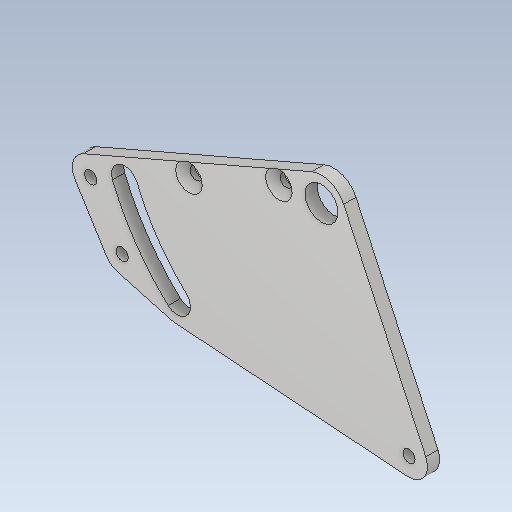
# Autodesk Inventor part: 中間外フレーム2
Saved by Autodesk Inventor 2020 (Build 240168000, 168)
## iProperties
Created: 2019-11-12
Part Number: 中間外フレーム2
Material: アルミニウム 2014-T4
Document SubType Name: Modeling
Designer: tanjihayato
Density: 2.8 g/cm^3
Appearance: サテン
Mass: 10.3329 g
Surface Area: 69.2935 cm^2
Volume: 3.69031 cm^3
Author: tanjihayato
Autodesk Inventor part; units mm, degrees
ref_plane "YZ Plane" through (0, 0, 0) normal (1, 0, 0) x (0, 1, 0)
ref_plane "XZ Plane" through (0, 0, 0) normal (0, 1, 0) x (-1, 0, 0)
ref_plane "XY Plane" through (0, 0, 0) normal (0, 0, 1) x (1, 0, 0)
sketch "スケッチ1" plane through (0, 0, 0) normal (0, 0, 1) x (1, 0, 0)
  circle A0 centre (0, 0) radius 20.55 construction
  circle A1 centre (-21.6908, -16.4118) radius 19.1 construction
  circle A2 centre (25.3202, -9.9362) radius 19.1 construction
  circle A3 centre (-50.601, 30.8143) radius 1.5
  circle A4 centre (5.9362, 53.5882) radius 1.5
  circle A5 centre (27.3908, 10.6821) radius 1.5
  circle A6 centre (-42.8914, 18.3887) radius 1.5
  circle A7 centre (-21.6908, -16.4118) radius 4.025
  circle A8 centre (25.3202, -9.9362) radius 4.025
  circle A9 centre (0, 0) radius 4
  line L0 (-17.8785, -18.8026) -> (-30.4168, -38.7963) construction
  arc A10 (-17.8785, -18.8026) -> (-19.2493, -12.6317) centre (-21.6908, -16.4118) ccw construction
  line L1 (-19.2493, -12.6317) -> (-39.0737, 0.1727) construction
  line L2 (37.1409, -30.8522) -> (21.8866, -12.8448) construction
  arc A11 (22.3659, -6.5417) -> (21.8866, -12.8448) centre (25.3202, -9.9362) ccw construction
  line L3 (22.3659, -6.5417) -> (40.1678, 8.9519) construction
  line L4 (-21.6908, -16.4118) -> (-99.9742, 13.5882) construction
  line L5 (-105.5257, -16.4118) -> (-21.6908, -16.4118) construction
  line L6 (-21.6908, -16.4118) -> (-101.7113, -41.4118) construction
  line L7 (25.3202, -9.9362) -> (102.5386, -46.4118) construction
  line L8 (110.4743, -16.4118) -> (25.3202, -9.9362) construction
  line L9 (25.3202, -9.9362) -> (108.6869, 8.5882) construction
  line L10 (-18.0583, -13.7557) -> (-31.9879, 5.2949) construction
  line L11 (-17.339, -17.5569) -> (-24.5367, -44.9106) construction
  line L12 (21.5077, -7.5456) -> (34.045, 12.4488) construction
  line L13 (21.0739, -11.4259) -> (31.6059, -41.446) construction
  arc A12 (-24.6176, -40.3201) -> (-19.5065, -44.4166) centre (-20.132, -39.9603) ccw
  circle A13 centre (-20.132, -39.9603) radius 3 construction
  arc A14 (-38.9879, 7.9907) -> (-39.3359, 8.5262) centre (-35.3982, 10.7044) ccw construction
  circle A15 centre (-35.3982, 10.7044) radius 3 construction
  arc A16 (-31.9879, 5.2949) -> (-33.8465, 6.7744) centre (-35.6204, 2.6388) ccw construction
  circle A17 centre (-41.5152, -3.6073) radius 1.5
  line L14 (-33.8465, 6.7744) -> (-56.066, 16.3055) construction
  line L15 (-41.3386, 0.8892) -> (-72.6317, 2.1181) construction
  circle A18 centre (-42.8914, 18.3887) radius 3 construction
  circle A19 centre (-35.3982, 10.7044) radius 1.5
  circle A20 centre (36.7736, 17.5344) radius 1.5
  arc A21 (40.7942, 15.5132) -> (40.1934, 20.4593) centre (36.7736, 17.5344) ccw
  circle A22 centre (25.6508, -33.5339) radius 1.5
  arc A23 (26.2763, -37.9902) -> (30.1508, -33.5178) centre (25.6508, -33.5339) ccw
  circle A24 centre (36.7736, 17.5344) radius 3 construction
  circle A25 centre (25.6508, -33.5339) radius 3 construction
  arc A26 (36.6836, 14.4025) -> (34.045, 12.4488) centre (37.8575, 10.0583) ccw construction
  line L16 (36.6836, 14.4025) -> (64.1968, 21.8369) construction
  line L17 (43.2599, 10.0553) -> (82.9273, 8.8396) construction
  circle A27 centre (27.3908, 10.6821) radius 3 construction
  circle A28 centre (-21.6908, -16.4118) radius 7.025 construction
  circle A29 centre (25.3202, -9.9362) radius 7.025 construction
  arc A30 (40.8593, 15.6483) -> (30.1508, -33.5178) centre (146.4685, -33.1029) ccw
  arc A31 (-24.6176, -40.3201) -> (-39.1827, 8.2484) centre (-145.1158, -49.988) ccw
  arc A32 (-52.2824, 34.9884) -> (-54.1907, 28.1005) centre (-50.601, 30.8143) ccw
  arc A33 (9.356, 56.5132) -> (4.2549, 57.7623) centre (5.9362, 53.5882) ccw
  line L18 (-39.1827, 8.2484) -> (-54.1907, 28.1005)
  line L19 (-52.2824, 34.9884) -> (4.2549, 57.7623)
  line L20 (9.356, 56.5132) -> (40.1934, 20.4593)
  line L21 (-19.5065, -44.4166) -> (26.2763, -37.9902)
  circle A34 centre (-20.132, -39.9603) radius 1.5
  line L22 (-23.8868, -42.4405) -> (-17.339, -17.5569)
  arc A35 (-17.339, -17.5569) -> (-18.0583, -13.7557) centre (-21.6908, -16.4118) ccw
  line L23 (-18.0583, -13.7557) -> (-31.9879, 5.2949)
  arc A36 (-31.9879, 5.2949) -> (-33.8465, 6.7744) centre (-35.6204, 2.6388) ccw
  line L24 (-33.8465, 6.7744) -> (-40.0946, 9.4545)
  line L25 (40.7974, 15.5141) -> (36.6836, 14.4025)
  arc A37 (36.6836, 14.4025) -> (34.045, 12.4488) centre (37.8575, 10.0583) ccw
  line L26 (34.045, 12.4488) -> (21.5077, -7.5456)
  arc A38 (21.5077, -7.5456) -> (21.0739, -11.4259) centre (25.3202, -9.9362) ccw
  line L27 (21.0739, -11.4259) -> (29.592, -35.7057)
  dimension "d0" = 8.05
  dimension "d1" = 8.05
  dimension "d2" = 8
  dimension "d3" = 20.968
  dimension "d4" = 20.968
  dimension "d5" = 17.35
  dimension "d6" = 17.35
  dimension "d7" = 16.877
  dimension "d8" = 16.877
  dimension "d9" = 20.936
  dimension "d10" = 20.936
  dimension "d11" = 9
  dimension "d12" = 6
  dimension "d13" = 9
  dimension "d14" = 6
  dimension "d15" = 9
  dimension "d16" = 20.968
  dimension "d17" = 20.968
  dimension "d18" = 6
  dimension "d19" = 3
  dimension "d20" = 3
  dimension "d21" = 9
  dimension "d22" = 3
  dimension "d23" = 9
  dimension "d24" = 6
  dimension "d25" = 6
  dimension "d26" = 9
  dimension "d27" = 16.877
  dimension "d28" = 3
  dimension "d29" = 3
  dimension "d30" = 9
  dimension "d31" = 9
  dimension "d32" = 3
  constraints: 56 end point, 40 point on circle, 39 centre point, 31 tangent, 14 coincident, 6 point on line, 2 equal length, 1 collinear, 1 concentric
  measures "d0" diameter of A7
  measures "d1" diameter of A8
  measures "d2" diameter of A9
  measures "d3" angle of L5 L4
  measures "d4" angle of L1 L10
  measures "d5" angle of L5 L6
  measures "d6" angle of L0 L11
  measures "d7" angle of L8 L9
  measures "d8" angle of L12 L3
  measures "d9" angle of L8 L7
  measures "d10" angle of L13 L2
  measures "d11" diameter of A12
  measures "d12" diameter of A13
  measures "d13" diameter of A14
  measures "d14" diameter of A15
  measures "d15" diameter of A16
  measures "d17" angle of L15 L14
  measures "d18" diameter of A18
  measures "d19" diameter of A19
  measures "d20" diameter of A20
  measures "d21" diameter of A21
  measures "d22" diameter of A22
  measures "d23" diameter of A23
  measures "d24" diameter of A24
  measures "d25" diameter of A25
  measures "d26" diameter of A26
  measures "d27" angle of L16 L17
  measures "d28" radial gap between concentric circles of A7 A28
  measures "d29" radial gap between concentric circles of A8 A29
  measures "d30" diameter of A32
  measures "d31" diameter of A33
  measures "d32" diameter of A34
sketch "スケッチ2" plane through (0, 0, 0) normal (0, 0, 1) x (1, 0, 0)
  circle A0 centre (-50.601, 30.8143) radius 1.5 projected
  circle A1 centre (-42.8914, 18.3887) radius 1.5 projected
  circle A2 centre (5.9362, 53.5882) radius 1.5 projected
  circle A3 centre (27.3908, 10.6821) radius 1.5 projected
  arc A4 (-52.3846, 34.9457) -> (-54.4248, 28.4418) centre (-50.601, 30.8143) ccw
  arc A5 (-46.7151, 16.0162) -> (-43.3819, 13.9155) centre (-42.8914, 18.3887) ccw
  arc A6 (11.384, 56.1025) -> (3.5581, 59.0968) centre (5.9362, 53.5882) ccw
  arc A7 (26.9003, 6.2089) -> (31.4766, 12.5678) centre (27.3908, 10.6821) ccw
  line L0 (-46.7151, 16.0162) -> (-54.4248, 28.4418)
  line L1 (-52.3846, 34.9457) -> (3.5581, 59.0968)
  line L2 (11.384, 56.1025) -> (31.4766, 12.5678)
  line L3 (26.9003, 6.2089) -> (-43.3819, 13.9155)
  circle A8 centre (5.9362, 53.5882) radius 4.025
  point P0 (0, 0)
  dimension "d33" = 3
  dimension "d34" = 3
  dimension "d35" = 4.5
  dimension "d36" = 3
  dimension "d39" = 8.05
  constraints: 8 end point, 8 point on circle, 8 tangent, 5 centre point, 1 coincident
  measures "d33" radial gap between concentric circles of A0 A4
  measures "d34" radial gap between concentric circles of A1 A5
  measures "d35" radial gap between concentric circles of A2 A6
  measures "d36" radial gap between concentric circles of A3 A7
  measures "d39" diameter of A8
extrude "押し出し1" add sketch "スケッチ2" along normal blind 3 contours L1 A6 L2 A7 L3 A5 L0 A4
sketch "スケッチ3" plane through (0, 0, 3) normal (0, 0, 1) x (1, 0, 0)
  circle A0 centre (5.9362, 53.5882) radius 4.025 projected
  circle A1 centre (27.3908, 10.6821) radius 1.5 projected
  circle A2 centre (-42.8914, 18.3887) radius 1.5 projected
  circle A3 centre (-50.601, 30.8143) radius 1.5 projected
  line L0 (-54.4248, 28.4418) -> (-46.7151, 16.0162) projected
  arc A4 (-46.7151, 16.0162) -> (-43.3819, 13.9155) centre (-42.8914, 18.3887) ccw projected
  line L1 (-43.3819, 13.9155) -> (26.9003, 6.2089) projected
  arc A5 (26.9003, 6.2089) -> (31.4766, 12.5678) centre (27.3908, 10.6821) ccw projected
  line L2 (31.4766, 12.5678) -> (11.384, 56.1025) projected
  arc A6 (11.384, 56.1025) -> (3.5581, 59.0968) centre (5.9362, 53.5882) ccw projected
  line L3 (3.5581, 59.0968) -> (-52.3846, 34.9457) projected
  arc A7 (-52.3846, 34.9457) -> (-54.4248, 28.4418) centre (-50.601, 30.8143) ccw projected
  circle A8 centre (5.9362, 53.5882) radius 6
  circle A9 centre (-26.5254, 42.8418) radius 1.5
  circle A10 centre (-4.491, 52.3543) radius 1.5
  circle A11 centre (-4.491, 52.3543) radius 4.5 construction
  point P0 (0, 0)
  dimension "d40" = 12
  dimension "d41" = 3
  dimension "d42" = 3
  dimension "d43" = 3
  dimension "d44" = 3
  dimension "d45" = 24
  dimension "d46" = 9
  constraints: 4 centre point, 2 coincident, 1 tangent
  measures "d40" diameter of A8
  measures "d41" diameter of A9
  measures "d42" diameter of A10
  measures "d43" distance from line of L3 A10.centre
  measures "d44" distance from line of L3 A9.centre
  measures "d45" distance of A9.centre A10.centre
  measures "d46" diameter of A11
extrude "押し出し2" cut sketch "スケッチ3" against normal blind 10 contours A9 | A10
chamfer "面取り1" distance 1.75 angle 45 2 edges at (-5.991, 52.3543, 3) (-28.0254, 42.8418, 3)
sketch "スケッチ4" plane through (0, 0, 3) normal (0, 0, 1) x (1, 0, 0)
  circle A0 centre (127.6431, 30.2622) radius 1.5
  circle A1 centre (5.9362, 53.5882) radius 1.5
  line L0 (5.9362, 53.5882) -> (127.6431, 30.2622) construction
  circle A2 centre (5.9362, 53.5882) radius 4.025
  circle A3 centre (127.6431, 30.2622) radius 4.025
  arc A4 (127.2517, 23.2481) -> (128.9655, 37.1616) centre (127.6431, 30.2622) ccw
  line L1 (12.8357, 52.2659) -> (13.4004, 55.2122)
  line L2 (15.4628, 54.817) -> (26.0698, 52.7841)
  line L3 (28.1322, 52.3888) -> (27.5675, 49.4424)
  line L4 (14.8981, 51.8706) -> (25.5051, 49.8377)
  line L5 (120.7437, 31.5845) -> (121.3084, 34.5309)
  line L6 (119.246, 34.9262) -> (108.639, 36.9591)
  line L7 (106.5765, 37.3543) -> (106.0119, 34.408)
  line L8 (108.0743, 34.0127) -> (118.6813, 31.9798)
  circle A5 centre (19.3546, 46.4346) radius 3
  circle A6 centre (112.5307, 28.5767) radius 3
  line L9 (7.2586, 60.4876) -> (128.9655, 37.1616)
  arc A7 (17.9263, 42.1672) -> (21.5465, 42.5045) centre (19.3546, 46.4346) ccw
  arc A8 (109.041, 25.7356) -> (112.28, 24.0837) centre (112.5307, 28.5767) ccw
  line L10 (3.7066, 46.9264) -> (17.9263, 42.1672)
  line L11 (112.28, 24.0837) -> (127.2517, 23.2481)
  circle A9 centre (19.3546, 46.4346) radius 1.5
  circle A10 centre (112.5307, 28.5767) radius 1.5
  line L12 (32.3442, 48.5269) -> (21.5465, 42.5045)
  line L13 (109.041, 25.7356) -> (101.2351, 35.3235)
  line L14 (32.3442, 48.5269) -> (101.2351, 35.3235)
  arc A11 (108.639, 36.9591) -> (106.5765, 37.3543) centre (107.6078, 37.1567) ccw
  arc A12 (106.0119, 34.408) -> (108.0743, 34.0127) centre (107.0431, 34.2103) ccw
  arc A13 (121.3084, 34.5309) -> (119.246, 34.9262) centre (120.2772, 34.7285) ccw
  arc A14 (118.6813, 31.9798) -> (120.7437, 31.5845) centre (119.7125, 31.7821) ccw
  arc A15 (28.1322, 52.3888) -> (26.0698, 52.7841) centre (27.101, 52.5864) ccw
  arc A16 (25.5051, 49.8377) -> (27.5675, 49.4424) centre (26.5363, 49.64) ccw
  arc A17 (15.4628, 54.817) -> (13.4004, 55.2122) centre (14.4316, 55.0146) ccw
  arc A18 (12.8357, 52.2659) -> (14.8981, 51.8706) centre (13.8669, 52.0682) ccw
  line L15 (5.9362, 53.5882) -> (-35.9404, 22.842) construction
  circle A19 centre (-35.9404, 22.842) radius 1.5
  arc A20 (-37.7159, 25.2602) -> (-34.165, 20.4238) centre (-35.9404, 22.842) ccw
  line L16 (-37.7159, 25.2602) -> (-0.9595, 52.247)
  line L17 (-34.165, 20.4238) -> (2.5914, 47.4106)
  arc A21 (7.2586, 60.4876) -> (-0.9595, 52.247) centre (5.9362, 53.5882) ccw
  arc A22 (2.5914, 47.4106) -> (3.7066, 46.9264) centre (5.9362, 53.5882) ccw
  circle A23 centre (0, 0) radius 10.1 construction
  circle A24 centre (25.3202, -9.9362) radius 17.1 construction
  circle A25 centre (110.4743, -16.4118) radius 28.1 construction
  circle A26 centre (62.4131, -12.7569) radius 20.1 construction
  circle A27 centre (-21.6908, -16.4118) radius 17.1 construction
  circle A28 centre (-105.5257, -16.4118) radius 28.1 construction
  line L18 (-170.915, -81.4118) -> (490.0044, -81.4118)
  line L19 (-105.5257, -16.4118) -> (-21.6908, -16.4118) construction
  line L20 (110.4743, -16.4118) -> (25.3202, -9.9362) construction
  line L21 (110.4743, -16.4118) -> (104.1501, -0.632)
  line L22 (104.1501, -0.632) -> (95.5937, 20.7173) construction
  line L23 (95.5937, 20.7173) -> (70.4743, -10.4118) construction
  line L24 (70.4743, -10.4118) -> (110.4743, -16.4118) construction
  line L25 (-137.6819, 53.5882) -> (165.8186, 53.5882)
  line L26 (25.3202, -9.9362) -> (108.6869, 8.5882) construction
  line L27 (25.3202, -9.9362) -> (102.5386, -46.4118) construction
  line L28 (25.3202, -9.9362) -> (5.9362, 53.5882) construction
  line L29 (5.9362, 53.5882) -> (127.6431, 30.2622)
  line L30 (127.6431, 30.2622) -> (110.4743, -16.4118) construction
  line L31 (102.5386, -46.4118) -> (118.0681, 0.8329) construction
  line L32 (118.0681, 0.8329) -> (5.9362, 53.5882) construction
  line L33 (108.6869, 8.5882) -> (129.8583, 53.5882) construction
  line L34 (129.8583, 53.5882) -> (5.9362, 53.5882) construction
  line L35 (119.2726, 31.0882) -> (366.4441, 68.5882) construction
  line L36 (119.0587, 6.9252) -> (362.0213, 65.8249) construction
  line L37 (110.3034, -22.7894) -> (351.0624, 44.5537) construction
  line L38 (127.6431, 30.2622) -> (4.1927, 19.4617) construction
  circle A29 centre (80.4743, 23.124) radius 3 construction
  circle A30 centre (80.4743, 23.124) radius 1.5
  arc A31 (79.801, 27.5733) -> (76.162, 24.4099) centre (80.4743, 23.124) ccw
  circle A32 centre (70.4743, -10.4118) radius 1.5
  arc A33 (66.162, -9.1259) -> (69.4242, -14.7876) centre (70.4743, -10.4118) ccw
  circle A34 centre (150.4743, 0.5882) radius 1.5
  arc A35 (152.5623, -3.3981) -> (154.0408, 3.3323) centre (150.4743, 0.5882) ccw
  circle A36 centre (127.6431, 30.2622) radius 1.5
  arc A37 (131.2816, 32.9102) -> (126.9698, 34.7115) centre (127.6431, 30.2622) ccw
  circle A38 centre (110.4743, -16.4118) radius 5
  arc A39 (108.6075, -24.1909) -> (114.1862, -23.4986) centre (110.4743, -16.4118) ccw
  line L39 (76.162, 24.4099) -> (66.162, -9.1259)
  line L40 (69.4242, -14.7876) -> (108.6075, -24.1909)
  line L41 (114.1862, -23.4986) -> (152.5623, -3.3981)
  line L42 (154.0408, 3.3323) -> (131.2097, 33.0062)
  line L43 (126.9698, 34.7115) -> (79.801, 27.5733)
  circle A40 centre (-145.5257, 0.5882) radius 1.5
  arc A41 (-149.0922, 3.3323) -> (-147.6136, -3.3981) centre (-145.5257, 0.5882) ccw
  circle A42 centre (-105.5257, -16.4118) radius 5
  arc A43 (-109.2375, -23.4986) -> (-103.6588, -24.1909) centre (-105.5257, -16.4118) ccw
  circle A44 centre (-65.5257, -10.4118) radius 1.5
  arc A45 (-64.4756, -14.7876) -> (-61.2133, -9.1259) centre (-65.5257, -10.4118) ccw
  circle A46 centre (0, 0) radius 20.05 construction
  circle A47 centre (110.4743, -16.4118) radius 30.1 construction
  circle A48 centre (62.4131, -12.7569) radius 22.1 construction
  circle A49 centre (25.3202, -9.9362) radius 19.1 construction
  circle A50 centre (0, 0) radius 12.1 construction
  circle A51 centre (-21.6908, -16.4118) radius 19.1 construction
  circle A52 centre (-105.5257, -16.4118) radius 30.1 construction
  circle A53 centre (0, 0) radius 20.55 construction
  circle A54 centre (95.5937, 20.7173) radius 4.025 construction
  circle A55 centre (95.5937, 20.7173) radius 6.025 construction
  circle A56 centre (-75.5257, 23.124) radius 1.5
  arc A57 (-71.2133, 24.4099) -> (-74.8523, 27.5733) centre (-75.5257, 23.124) ccw
  circle A58 centre (-122.6945, 30.2622) radius 1.5
  arc A59 (-122.0212, 34.7115) -> (-126.261, 33.0062) centre (-122.6945, 30.2622) ccw
  line L44 (-126.261, 33.0062) -> (-149.0922, 3.3323)
  line L45 (-147.6136, -3.3981) -> (-109.2375, -23.4986)
  line L46 (-103.6588, -24.1909) -> (-64.4756, -14.7876)
  line L47 (-61.2133, -9.1259) -> (-71.2133, 24.4099)
  line L48 (-74.8523, 27.5733) -> (-122.0212, 34.7115)
  circle A60 centre (14, -17.4118) radius 2.2921 construction
  circle A61 centre (-14, -17.4118) radius 2.2921 construction
  circle A62 centre (-14, -17.4118) radius 14 construction
  circle A63 centre (14, -17.4118) radius 14 construction
  line L49 (-170.6512, -31.4118) -> (202.8656, -31.4118)
  line L50 (5.9362, 53.5882) -> (-42.2529, 34.177) construction
  line L51 (5.9362, 53.5882) -> (-29.4045, 15.5091) construction
  circle A64 centre (5.9362, 53.5882) radius 1.5
  arc A65 (9.9611, 55.6008) -> (4.2549, 57.7623) centre (5.9362, 53.5882) ccw
  line L52 (-21.6908, -16.4118) -> (-99.9742, 13.5882) construction
  line L53 (-21.6908, -16.4118) -> (-101.7113, -41.4118) construction
  line L54 (9.9611, 55.6008) -> (31.4156, 12.6947)
  circle A66 centre (-50.601, 30.8143) radius 1.5
  arc A67 (-52.2824, 34.9884) -> (-54.4248, 28.4418) centre (-50.601, 30.8143) ccw
  line L55 (4.2549, 57.7623) -> (-52.2824, 34.9884)
  line L56 (-54.4248, 28.4418) -> (-46.7151, 16.0162)
  circle A68 centre (27.3908, 10.6821) radius 3 construction
  circle A69 centre (-84.8661, 5.2713) radius 4.5 construction
  circle A70 centre (-132.0174, -1.9813) radius 4.5 construction
  line L57 (-132.7015, 2.4664) -> (-85.5502, 9.719) construction
  arc A71 (26.9003, 6.2089) -> (31.4156, 12.6947) centre (27.3908, 10.6821) ccw
  arc A72 (-46.7151, 16.0162) -> (-43.3819, 13.9155) centre (-42.8914, 18.3887) ccw
  line L58 (-43.3819, 13.9155) -> (26.9003, 6.2089)
  circle A73 centre (-42.2529, 34.177) radius 3 construction
  circle A74 centre (25.3202, -9.9362) radius 4.025 construction
  circle A75 centre (-21.6908, -16.4118) radius 4.025 construction
  circle A76 centre (-42.8914, 18.3887) radius 1.5
  circle A77 centre (27.3908, 10.6821) radius 1.5
  circle A78 centre (-57.813, 39.7705) radius 4.5 construction
  circle A79 centre (-99.304, 63.3152) radius 4.5 construction
  line L59 (5.9362, 53.5882) -> (-35.9404, 22.842) construction
  circle A80 centre (-58.0056, -24.4791) radius 20.1 construction
  circle A81 centre (-58.0056, -24.4791) radius 22.1 construction
  line L60 (-53.3261, 39.4281) -> (-56.2797, 0.7243) construction
  circle A82 centre (-42.2529, 34.177) radius 4.5
  dimension "d169" = 9
  dimension "d170" = 9
  dimension "d185" = 9
  dimension "d52" = 8.05
  dimension "d53" = 8.05
  dimension "d54" = 3
  dimension "d55" = 3
  dimension "d56" = 15
  dimension "d57" = 3
  dimension "d58" = 15
  dimension "d59" = 6
  dimension "d60" = 6
  dimension "d61" = 9
  dimension "d62" = 9
  dimension "d63" = 3
  dimension "d64" = 3
  dimension "d65" = 7.5
  dimension "d66" = 7.5
  dimension "d67" = 40
  dimension "d68" = 40
  dimension "d69" = 2.1
  dimension "d70" = 2.1
  dimension "d71" = 2.1
  dimension "d72" = 2.1
  dimension "d73" = 2.1
  dimension "d74" = 2.1
  dimension "d75" = 2.1
  dimension "d76" = 2.1
  dimension "d77" = 3
  dimension "d78" = 6
  dimension "d79" = 3
  dimension "d80" = 3
  dimension "d81" = 20.2
  dimension "d82" = 34.2
  dimension "d83" = 56.2
  dimension "d84" = 40.2
  dimension "d85" = 216
  dimension "d86" = 65
  dimension "d87" = 65
  dimension "d88" = 34.2
  dimension "d89" = 56.2
  dimension "d90" = 17
  dimension "d91" = 23
  dimension "d92" = 40
  dimension "d93" = 40
  dimension "d94" = 6
  dimension "d95" = 135
  dimension "d96" = 25
  dimension "d97" = 30
  dimension "d98" = 5
  dimension "d99" = 2
  dimension "d100" = 250
  dimension "d101" = 150
  dimension "d102" = 250
  dimension "d103" = 250
  dimension "d104" = 123.823
  dimension "d105" = 123.823
  dimension "d106" = 123.823
  dimension "d107" = 6
  dimension "d108" = 3
  dimension "d109" = 9
  dimension "d110" = 3
  dimension "d111" = 9
  dimension "d112" = 3
  dimension "d113" = 9
  dimension "d114" = 40
  dimension "d115" = 17
  constraints: 122 end point, 80 centre point, 61 tangent, 57 point on circle, 37 coincident, 17 point on line, 11 equal length, 5 horizontal, 5 parallel, 5 perpendicular, 3 midpoint, 2 collinear, 2 equal radius, 13 other
  measures "d52" diameter of A2
  measures "d53" diameter of A3
  measures "d54" radial gap between concentric circles of A3 A4
  measures "d55" distance of L1.start L1.end
  measures "d56" distance of L1.end L3.start
  measures "d57" distance of L5.start L5.end
  measures "d58" distance of L5.end L7.start
  measures "d59" diameter of A5
  measures "d60" diameter of A6
  measures "d61" diameter of A7
  measures "d62" diameter of A8
  measures "d63" diameter of A9
  measures "d64" diameter of A10
  measures "d65" distance from line of A5.centre L3
  measures "d66" distance from line of A10.centre L7
  measures "d67" angle of L13 L0
  measures "d68" angle of L0 L12
  measures "d69" diameter of A11
  measures "d70" diameter of A12
  measures "d71" diameter of A13
  measures "d72" diameter of A14
  measures "d73" diameter of A15
  measures "d74" diameter of A16
  measures "d75" diameter of A17
  measures "d76" diameter of A18
  measures "d77" diameter of A19
  measures "d78" diameter of A20
  measures "d79" radial gap between concentric circles of A21 A2
  measures "d80" radial gap between concentric circles of A22 A2
  measures "d81" diameter of A23
  measures "d82" diameter of A24
  measures "d83" diameter of A25
  measures "d84" diameter of A26
  measures "d85" distance of L19.start L20.start
  measures "d86" distance from line of L18 L20.start
  measures "d87" distance from line of L18 L19.start
  measures "d88" diameter of A27
  measures "d89" diameter of A28
  measures "d90" distance of L20.start L21.end
  measures "d91" distance of L21.end L22.end
  measures "d92" distance of L22.end L23.end
  measures "d93" horizontal distance of L23.end L20.start
  measures "d94" vertical distance of L23.end L20.start
  measures "d95" distance between parallel lines of L18 L25
  measures "d96" vertical distance of L20.start L26.end
  measures "d97" vertical distance of L27.end L20.start
  measures "d98" angle of L30 L33
  measures "d99" angle of L30 L31
  measures "d100" distance of L35.start L35.end
  measures "d101" distance from line of L18 L35.end
  measures "d102" distance of L36.start L36.end
  measures "d103" distance of L37.start L37.end
  measures "d104" angle of L33 L35
  measures "d105" angle of L30 L36
  measures "d106" angle of L31 L37
  measures "d107" diameter of A29
  measures "d108" diameter of A30
  measures "d109" diameter of A31
  measures "d110" diameter of A32
  measures "d111" diameter of A33
  measures "d112" diameter of A34
  measures "d113" diameter of A35
  measures "d114" horizontal distance of L20.start A34.centre
  measures "d115" vertical distance of L20.start A34.centre
sketch "スケッチ5" plane through (0, 0, 3) normal (0, 0, 1) x (1, 0, 0)
  arc A0 (-42.2529, 34.177) -> (-29.4045, 15.5091) centre (5.9362, 53.5882) ccw construction
  arc A1 (-45.2675, 32.9627) -> (-31.6153, 13.1269) centre (5.9362, 53.5882) ccw
  arc A2 (-39.2383, 35.3914) -> (-27.1936, 17.8913) centre (5.9362, 53.5882) ccw
  arc A3 (-39.2383, 35.3914) -> (-45.2675, 32.9627) centre (-42.2529, 34.177) ccw
  arc A4 (-31.6153, 13.1269) -> (-27.1936, 17.8913) centre (-29.4045, 15.5091) ccw
  arc A5 (-37.3831, 36.1386) -> (-25.8331, 19.3572) centre (5.9362, 53.5882) ccw
  arc A6 (-37.3831, 36.1386) -> (-47.1226, 32.2154) centre (-42.2529, 34.177) ccw
  arc A7 (-47.1226, 32.2154) -> (-32.9758, 11.661) centre (5.9362, 53.5882) ccw
  arc A8 (-28.862, 45.1007) -> (-26.5668, 46.0915) centre (-26.5254, 42.8418) ccw projected
  line L0 (-28.862, 45.1007) -> (-52.3846, 34.9457) projected
  arc A9 (-52.3846, 34.9457) -> (-54.4248, 28.4418) centre (-50.601, 30.8143) ccw projected
  line L1 (-54.4248, 28.4418) -> (-46.7151, 16.0162) projected
  arc A10 (-46.7151, 16.0162) -> (-43.3819, 13.9155) centre (-42.8914, 18.3887) ccw projected
  line L2 (-43.3819, 13.9155) -> (26.9003, 6.2089) projected
  arc A11 (26.9003, 6.2089) -> (31.4766, 12.5678) centre (27.3908, 10.6821) ccw projected
  line L3 (31.4766, 12.5678) -> (11.384, 56.1025) projected
  arc A12 (11.384, 56.1025) -> (3.5581, 59.0968) centre (5.9362, 53.5882) ccw projected
  line L4 (3.5581, 59.0968) -> (-4.5324, 55.604) projected
  arc A13 (-6.8277, 54.6131) -> (-4.5324, 55.604) centre (-4.491, 52.3543) ccw projected
  line L5 (-6.8277, 54.6131) -> (-26.5668, 46.0915) projected
  circle A14 centre (5.9362, 53.5882) radius 4.025 projected
  circle A15 centre (27.3908, 10.6821) radius 1.5 projected
  circle A16 centre (-42.8914, 18.3887) radius 1.5 projected
  circle A17 centre (-50.601, 30.8143) radius 1.5 projected
  arc A18 (-46.7151, 16.0162) -> (-43.3819, 13.9155) centre (-42.8914, 18.3887) ccw projected
  line L6 (-29.7802, 10.2726) -> (27.0687, 6.1936)
  arc A19 (26.9003, 6.2089) -> (31.4766, 12.5678) centre (27.3908, 10.6821) ccw projected
  line L7 (-44.0689, 14.0455) -> (-30.7783, 10.442)
  arc A20 (-30.7783, 10.442) -> (-29.7802, 10.2726) centre (-29.4045, 15.5091) ccw
  arc A21 (-25.537, 11.9588) -> (-25.8331, 19.3572) centre (-29.4045, 15.5091) ccw
  point P0 (0, 0)
  point P1 (-35.9404, 22.842)
  dimension "d199" = 6.5
  dimension "d200" = 2
  dimension "d201" = 2
  constraints: 23 point on circle, 10 centre point, 8 tangent, 4 end point, 1 point on line, 2 other
  measures "d199" diameter of A4
  measures "d200" radial gap between concentric circles of A2 A5
  measures "d201" radial gap between concentric circles of A20 A4
extrude "押し出し3" add sketch "スケッチ5" against normal blind 3 contours L2 A4 | A4 L2 A11 L6 A20 L7 A10
extrude "押し出し4" cut sketch "スケッチ5" against normal blind 3 contours A3 A2 A4 L2 A1 | L2 A4
sketch "スケッチ6" plane through (0, 0, 0) normal (0, 0, -1) x (-1, 0, 0)
  arc A0 (27.1936, 17.8913) -> (31.6153, 13.1269) centre (29.4045, 15.5091) ccw projected
  arc A1 (27.1936, 17.8913) -> (39.2383, 35.3914) centre (-5.9362, 53.5882) ccw projected
  arc A2 (45.2675, 32.9627) -> (39.2383, 35.3914) centre (42.2529, 34.177) ccw projected
  arc A3 (31.6153, 13.1269) -> (45.2675, 32.9627) centre (-5.9362, 53.5882) ccw projected
  circle A4 centre (26.5254, 42.8418) radius 1.5 projected
  circle A5 centre (4.491, 52.3543) radius 1.5 projected
  circle A6 centre (-5.9362, 53.5882) radius 4.025 projected
  circle A7 centre (-27.3908, 10.6821) radius 1.5 projected
  circle A8 centre (42.8914, 18.3887) radius 1.5 projected
  circle A9 centre (50.601, 30.8143) radius 1.5 projected
  line L0 (46.7151, 16.0162) -> (54.4248, 28.4418) projected
  arc A10 (54.4248, 28.4418) -> (52.3846, 34.9457) centre (50.601, 30.8143) ccw projected
  line L1 (52.3846, 34.9457) -> (-3.5581, 59.0968) projected
  arc A11 (-3.5581, 59.0968) -> (-11.384, 56.1025) centre (-5.9362, 53.5882) ccw projected
  line L2 (-11.384, 56.1025) -> (-31.4766, 12.5678) projected
  arc A12 (-31.4766, 12.5678) -> (-27.0687, 6.1936) centre (-27.3908, 10.6821) ccw projected
  line L3 (-27.0687, 6.1936) -> (29.7802, 10.2726) projected
  arc A13 (29.7802, 10.2726) -> (30.7783, 10.442) centre (29.4045, 15.5091) ccw projected
  line L4 (30.7783, 10.442) -> (44.0689, 14.0455) projected
  arc A14 (44.0689, 14.0455) -> (46.7151, 16.0162) centre (42.8914, 18.3887) ccw projected
  line L5 (-4.7472, 56.3425) -> (51.1956, 32.1914)
  arc A15 (51.8756, 30.0234) -> (51.1956, 32.1914) centre (50.601, 30.8143) ccw
  line L6 (51.8756, 30.0234) -> (44.166, 17.5978)
  arc A16 (43.2839, 16.9409) -> (44.166, 17.5978) centre (42.8914, 18.3887) ccw
  line L7 (43.2839, 16.9409) -> (29.9932, 13.3375)
  arc A17 (29.5655, 13.2649) -> (29.9932, 13.3375) centre (29.4045, 15.5091) ccw
  line L8 (29.5655, 13.2649) -> (-27.2834, 9.1859)
  arc A18 (-28.7527, 11.3107) -> (-27.2834, 9.1859) centre (-27.3908, 10.6821) ccw
  line L9 (-28.7527, 11.3107) -> (-8.6601, 54.8454)
  arc A19 (-4.7472, 56.3425) -> (-8.6601, 54.8454) centre (-5.9362, 53.5882) ccw
  arc A20 (-11.322, 49.0778) -> (0.3825, 50.5184) centre (-5.9362, 53.5882) ccw
  arc A21 (25.1528, 20.0902) -> (36.4555, 36.5123) centre (-5.9362, 53.5882) ccw
  arc A22 (25.1528, 20.0902) -> (23.7495, 12.8476) centre (29.4045, 15.5091) ccw
  arc A23 (33.6561, 10.928) -> (34.0975, 11.3419) centre (-5.9362, 53.5882) ccw
  arc A24 (22.3939, 44.6254) -> (30.6568, 41.0582) centre (26.5254, 42.8418) ccw
  arc A25 (0.3825, 50.5184) -> (8.6224, 50.5707) centre (4.491, 52.3543) ccw
  arc A26 (-23.0517, 9.4896) -> (-26.9748, 15.1628) centre (-27.3908, 10.6821) ccw
  arc A27 (37.419, 38.1389) -> (36.4555, 36.5123) centre (42.2529, 34.177) ccw
  point P0 (0, 0)
  dimension "d206" = 3
  dimension "d207" = 3
  dimension "d208" = 3
  dimension "d209" = 3
  dimension "d210" = 3
  dimension "d212" = 3
  dimension "d213" = 3
  dimension "d214" = 3
  constraints: 26 point on circle, 13 centre point, 10 end point, 9 point on line, 1 coincident, 9 other
  measures "d206" distance between parallel lines of L1 L5
  measures "d207" radial gap between concentric circles of A6 A20
  measures "d208" radial gap between concentric circles of A1 A21
  measures "d209" radial gap between concentric circles of A4 A24
  measures "d210" radial gap between concentric circles of A5 A25
  measures "d212" radial gap between concentric circles of A26 A7
  measures "d213" radial gap between concentric circles of A27 A2
  measures "d214" radial gap between concentric circles of A22 A0
extrude "押し出し5" cut sketch "スケッチ6" against normal blind 2.5 contours L8 A26 L9 A20 A25 L5 A24 A27 A21 A22
fillet "フィレット1" radius 1 9 edges at (-23.7495, 12.8476, 1.25) (23.0517, 9.4896, 1.25) (26.9748, 15.1628, 1.25) (11.322, 49.0778, 1.25) (-0.3825, 50.5184, 1.25) (-8.6224, 50.5707, 1.25) (-22.3939, 44.6254, 1.25) (-30.6568, 41.0582, 1.25) (-37.419, 38.1389, 1.25)
equation "\"d4\" = d3"
equation "\"d6\" = d5"
equation "\"d8\" = d7"
equation "\"d10\" = d9"
equation "\"d16\" = d3"
equation "\"d17\" = d3"
equation "\"d27\" = d7"
equation "\"d68\" = d67"
equation "\"d88\" = d82"
equation "\"d89\" = d83"
equation "\"d105\" = d104"
equation "\"d106\" = d104"
